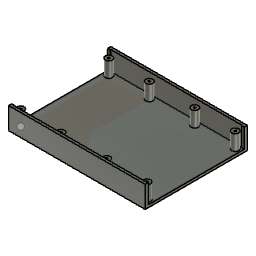
Boitier_sequenceur v3 (Autodesk Fusion 360 design; units mm, degrees)
Autodesk Fusion 360 part; units mm, degrees
sketch "Esquisse1" plane through (0, 0, 0) normal (0, 0, 1) x (1, 0, 0)
  line L0 (107, 80) -> (-107, 80)
  line L1 (-107, 80) -> (-107, -80)
  line L2 (-107, -80) -> (107, -80)
  line L3 (107, -80) -> (107, 80)
  line L4 (107, 80) -> (-107, -80) construction
  line L5 (-107, 80) -> (107, -80) construction
  dimension "d1" = 214
  constraint horizontal L0
  constraint perpendicular L0 L1
  constraint parallel L0 L2
  constraint parallel L1 L3
  constraint coincident L4 origin
  constraint coincident L5 origin
  measures "d1" distance of L1.end L2.end
extrude "Extrusion1" add sketch "Esquisse1" along normal blind 40
sketch "Esquisse2" plane through (0, 0, 40) normal (0, 0, 1) x (-1, 0, 0)
  line L0 (-107, 80) -> (-107, -80)
  line L1 (-107, -80) -> (107, -80)
  line L2 (107, -80) -> (107, 80)
  line L3 (107, 80) -> (-107, 80)
  line L4 (-103, 76) -> (-103, -76)
  line L5 (-103, -76) -> (103, -76)
  line L6 (103, -76) -> (103, 76)
  line L7 (103, 76) -> (-103, 76)
  dimension "d4" = -4
extrude "Extrusion2" cut sketch "Esquisse2" against normal blind 36 contours L4 L5 L6 L7
sketch "Esquisse3" plane through (0, 0, 4) normal (0, 0, 1) x (-1, 0, 0)
  line L0 (103, 76) -> (-103, 76)
  line L1 (-103, 76) -> (-103, -76)
  line L2 (-103, -76) -> (103, -76)
  line L3 (103, -76) -> (103, 76)
sketch "Esquisse4" plane through (0, 0, 4) normal (0, 0, 1) x (-1, 0, 0)
sketch "Esquisse5" plane through (0, 0, 4) normal (0, 0, 1) x (-1, 0, 0)
  circle A0 centre (99, -69) radius 5.5
  circle A1 centre (99, -69) radius 1.5
  dimension "d11" = 11
  dimension "d12" = -4
  measures "d11" diameter of A0
extrude "Extrusion3" add sketch "Esquisse5" along normal blind 34
sketch "Esquisse6" plane through (0, 0, 4) normal (0, 0, 1) x (-1, 0, 0)
  point P0 (99, 69)
sketch "Esquisse7" plane through (0, 0, 4) normal (0, 0, 1) x (-1, 0, 0)
  circle A0 centre (99, 69) radius 5.5
  dimension "d16" = 11
  measures "d16" diameter of A0
sketch "Esquisse8" plane through (0, 0, 4) normal (0, 0, 1) x (1, 0, 0)
sketch "Esquisse9" plane through (0, 0, 4) normal (0, 0, 1) x (1, 0, 0)
sketch "Esquisse10" plane through (0, 0, 4) normal (0, 0, 1) x (1, 0, 0)
extrude "Extrusion4" add sketch "Esquisse7" along normal blind 34
sketch "Esquisse11" plane through (0, 0, 38) normal (0, 0, 1) x (-1, 0, 0)
  line L0 (103, 65.2251) -> (103, 72.7749)
  arc A0 (103, 72.7749) -> (103, 65.2251) centre (99, 69) ccw
sketch "Esquisse12" plane through (0, 0, 38) normal (0, 0, 1) x (-1, 0, 0)
sketch "Esquisse13" plane through (0, 0, 38) normal (0, 0, 1) x (1, 0, 0)
sketch "Esquisse14" plane through (0, 0, 38) normal (0, 0, 1) x (-1, 0, 0)
  circle A0 centre (99, 69) radius 1.5
  dimension "d19" = 3
  measures "d19" diameter of A0
extrude "Extrusion5" cut sketch "Esquisse14" against normal blind 34
sketch "Esquisse15" plane through (0, 0, 4) normal (0, 0, 1) x (-1, 0, 0)
  circle A0 centre (-99, -69) radius 5.5
  circle A1 centre (-99, 69) radius 5.5
  dimension "d23" = 11
  dimension "d24" = 11
  measures "d23" diameter of A0
  measures "d24" diameter of A1
extrude "Extrusion6" add sketch "Esquisse15" along normal blind 34 contours A1
sketch "Esquisse16" plane through (0, 0, 4) normal (0, 0, 1) x (-1, 0, 0)
  circle A0 centre (-99, -69) radius 5.5
  dimension "d28" = 11
  measures "d28" diameter of A0
extrude "Extrusion7" add sketch "Esquisse16" along normal blind 34
sketch "Esquisse17" plane through (0, 0, 38) normal (0, 0, 1) x (-1, 0, 0)
  line L0 (-103, -65.2251) -> (-103, -72.7749)
  arc A0 (-103, -72.7749) -> (-103, -65.2251) centre (-99, -69) ccw
  circle A1 centre (-99, -69) radius 1.5
  dimension "d31" = 3
  constraint concentric A0 A1
  measures "d31" diameter of A1
extrude "Extrusion8" cut sketch "Esquisse17" against normal blind 34 contours A1
sketch "Esquisse18" plane through (0, 0, 38) normal (0, 0, 1) x (-1, 0, 0)
  line L0 (-103, 72.7749) -> (-103, 65.2251)
  arc A0 (-103, 65.2251) -> (-103, 72.7749) centre (-99, 69) ccw
  circle A1 centre (-99, 69) radius 1.5
  dimension "d34" = 3
  constraint concentric A0 A1
  measures "d34" diameter of A1
extrude "Extrusion9" cut sketch "Esquisse18" against normal blind 34 contours A1
sketch "Esquisse19" plane through (-107, 0, 0) normal (-1, 0, 0) x (0, -1, 0)
  line L0 (-80, 0) -> (80, 0)
  line L1 (80, 0) -> (80, 40)
  line L2 (80, 40) -> (-80, 40)
  line L3 (-80, 40) -> (-80, 0)
  line L4 (-75, 40) -> (75, 40)
  line L5 (75, 40) -> (75, 4)
  line L6 (75, 4) -> (-75, 4)
  line L7 (-75, 4) -> (-75, 40)
  dimension "d37" = 36
  constraint horizontal L4
  constraint vertical L5
  constraint horizontal L6
  constraint vertical L7
  constraint coincident L2 L4.start
  measures "d37" distance of L4 L6
extrude "Extrusion10" cut sketch "Esquisse19" against normal blind 4 contours L2 L4 L5 L6 L7
sketch "Esquisse20" plane through (107, 0, 0) normal (1, 0, 0) x (0, 1, 0)
  line L0 (-80, 0) -> (80, 0)
  line L1 (80, 0) -> (80, 40)
  line L2 (80, 40) -> (-80, 40)
  line L3 (-80, 40) -> (-80, 0)
  line L4 (-75, 40) -> (75, 40)
  line L5 (75, 40) -> (75, 4)
  line L6 (75, 4) -> (-75, 4)
  line L7 (-75, 4) -> (-75, 40)
  dimension "d40" = 36
  constraint horizontal L4
  constraint vertical L5
  constraint horizontal L6
  constraint vertical L7
  constraint coincident L2 L4.start
  measures "d40" distance of L4 L6
extrude "Extrusion11" cut sketch "Esquisse20" against normal blind 4 contours L2 L4 L5 L6 L7
extrude "Extrusion12" cut 2 faces at (-34.3333, 78.6667, 40) (34.3333, -78.6667, 40) along direction (0, 0, -1) blind 10
extrude "Extrusion13" cut sketch "Esquisse11" 3 faces at (-102.1667, 69, 38) (102.1667, 69, 38) (102.1667, -69, 38) against normal blind 10
sketch "Esquisse21" plane through (0, 0, 28) normal (0, 0, 1) x (-1, 0, 0)
  circle A0 centre (-99, -69) radius 1.5
  line L0 (-103, -65.2251) -> (-103, -72.7749)
  arc A1 (-103, -72.7749) -> (-103, -65.2251) centre (-99, -69) ccw
  circle A2 centre (-99, -69) radius 5.5
  constraint concentric A0 A2
extrude "Extrusion14" add sketch "Esquisse21" against normal blind 24 contours L0 A2
sketch "Esquisse22" plane through (0, 0, 28) normal (0, 0, 1) x (-1, 0, 0)
  circle A0 centre (-99, 69) radius 1.5
  line L0 (-103, 72.7749) -> (-103, 65.2251)
  arc A1 (-103, 65.2251) -> (-103, 72.7749) centre (-99, 69) ccw
  circle A2 centre (-99, 69) radius 5.5
  constraint concentric A0 A2
extrude "Extrusion15" add sketch "Esquisse22" against normal blind 24 contours L0 A2
sketch "Esquisse23" plane through (0, 0, 28) normal (0, 0, 1) x (-1, 0, 0)
  circle A0 centre (99, 69) radius 1.5
  arc A1 (103, 72.7749) -> (103, 65.2251) centre (99, 69) ccw
  line L0 (103, 65.2251) -> (103, 72.7749)
  circle A2 centre (99, 69) radius 5.5
  constraint concentric A0 A2
extrude "Extrusion16" add sketch "Esquisse23" against normal blind 24 contours L0 A2
sketch "Esquisse24" plane through (0, 0, 28) normal (0, 0, 1) x (-1, 0, 0)
  line L0 (103, -72.7749) -> (103, -65.2251)
  arc A0 (103, -65.2251) -> (103, -72.7749) centre (99, -69) ccw
  circle A1 centre (99, -69) radius 1.5
  circle A2 centre (99, -69) radius 5.5
  constraint concentric A0 A2
  constraint coincident L0.end A2
extrude "Extrusion17" add sketch "Esquisse24" against normal blind 24 contours L0 A2
sketch "Esquisse25" plane through (0, 0, 4) normal (0, 0, 1) x (-1, 0, 0)
  circle A0 centre (-35.66, 69) radius 5.5
  circle A1 centre (35.66, 69) radius 5.5
  circle A2 centre (35.66, -69) radius 5.5
  circle A3 centre (-35.66, -69) radius 5.5
  dimension "d56" = 11
  dimension "d57" = 11
  dimension "d58" = 11
  dimension "d59" = 11
  measures "d56" diameter of A0
  measures "d57" diameter of A1
  measures "d58" diameter of A2
  measures "d59" diameter of A3
extrude "Extrusion18" add sketch "Esquisse25" along normal blind 24
extrude "Extrusion19" add 2 faces at (-34.3333, 78.6667, 30) (34.3333, -78.6667, 30) along direction (0, 0, 1) blind 4
sketch "Esquisse26" plane through (0, 0, 28) normal (0, 0, 1) x (-1, 0, 0)
  circle A0 centre (-35.66, -69) radius 5.5
  circle A1 centre (-35.66, -69) radius 1.5
  dimension "d64" = 3
  constraint concentric A0 A1
  measures "d64" diameter of A1
sketch "Esquisse27" plane through (0, 0, 28) normal (0, 0, 1) x (-1, 0, 0)
  circle A0 centre (-35.66, 69) radius 5.5
  circle A1 centre (-35.66, 69) radius 1.5
  dimension "d65" = 3
  constraint concentric A0 A1
  measures "d65" diameter of A1
sketch "Esquisse28" plane through (0, 0, 28) normal (0, 0, 1) x (-1, 0, 0)
  circle A0 centre (35.66, 69) radius 5.5
  circle A1 centre (35.66, 69) radius 1.5
  dimension "d66" = 3
  constraint concentric A0 A1
  measures "d66" diameter of A1
sketch "Esquisse29" plane through (0, 0, 28) normal (0, 0, 1) x (-1, 0, 0)
  circle A0 centre (35.66, -69) radius 5.5
  circle A1 centre (35.66, -69) radius 1.5
  dimension "d67" = 3
  constraint concentric A0 A1
  measures "d67" diameter of A1
extrude "Extrusion20" cut sketch "Esquisse28" sketch "Esquisse29" sketch "Esquisse26" sketch "Esquisse27" against normal blind 24 contours A1 of sketch 2 contours A1 of sketch 3 contours A1 of sketch 4 contours A1
